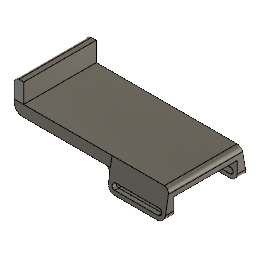
laptop_slider (Autodesk Fusion 360 design; units mm, degrees)
Autodesk Fusion 360 part; units mm, degrees
sketch "Sketch1" plane through (0, 0, 0) normal (0, 0, 1) x (1, 0, 0)
  line L0 (160, 0) -> (160, 10)
  line L1 (160, 10) -> (10, 10)
  line L2 (0, 10) -> (0, 25)
  line L3 (5, 30) -> (10, 30)
  line L4 (10, 30) -> (10, 10)
  arc A0 (5, 30) -> (0, 25) centre (5, 25) ccw
  line L5 (146, 0) -> (146, -12.5)
  line L6 (160, -12.5) -> (160, 0)
  arc A1 (146, -12.5) -> (160, -12.5) centre (153, -12.5) ccw
  line L7 (101, -12.5) -> (101, 0)
  line L8 (115, -12.5) -> (115, 0)
  arc A2 (101, -12.5) -> (115, -12.5) centre (108, -12.5) ccw
  line L9 (10, 0) -> (101, 0)
  line L10 (115, 0) -> (146, 0)
  line L11 (108, -15.5) -> (109.157, -15.2679)
  line L12 (153.0016, -15.5) -> (108, -15.5)
  line L13 (108, -9.5) -> (153, -9.5)
  line L14 (153, -19.5) -> (108, -19.5)
  arc A3 (108, -9.5) -> (109.157, -15.2679) centre (108, -12.5) ccw
  arc A4 (153.0016, -15.5) -> (153, -9.5) centre (153, -12.5) ccw
  arc A5 (0, 10) -> (10, 0) centre (10, 10) ccw
  point P0 (0, 30)
  dimension "d1" = 160
  dimension "d2" = 10
  dimension "d3" = 20
  dimension "d4" = 10
  dimension "d6" = 5
  dimension "d7" = 25
  dimension "d8" = 6
  dimension "d10" = 14
  dimension "d12" = 6
  dimension "d14" = 14
  dimension "d15" = 22.5
  dimension "d16" = 14
  dimension "d31" = 45
  dimension "d45" = 10
  constraint horizontal L9
  constraint vertical L0
  constraint horizontal L1
  constraint perpendicular L1 L2
  constraint perpendicular L2 L3
  constraint perpendicular L1 L4
  constraint coincident origin L9
  constraint coincident P0 L2
  constraint coincident P0 L3
  constraint tangent L2 A0
  constraint tangent L3 A0
  constraint concentric A1 A4
  constraint coincident L5.start L9
  constraint tangent L5 A1
  constraint coincident L0.start L9
  constraint tangent L6 A1
  constraint perpendicular L6 L9
  constraint concentric A2 A3
  constraint perpendicular L7 L9
  constraint coincident L8.end L9
  constraint perpendicular L8 L9
  constraint collinear L9 L10
  constraint coincident L11.start A3
  constraint horizontal L12
  constraint coincident L13.end A4
  constraint tangent L13 A4
  constraint midpoint A1 L14.start
  constraint midpoint A2 L14.end
  constraint coincident L13 A4.end
  constraint tangent L13 A3
  constraint tangent L12 A3
  constraint coincident L0.start L6.end
  constraint tangent L2 A5
  constraint tangent L9 A5
  measures "d1" distance of origin L0.start
  measures "d2" distance of L0.start L0.end
  measures "d3" distance of L2.start P0
  measures "d4" distance of P0 L3.end
  measures "d6" radius of A0
  measures "d7" distance of A0.centre L9
  measures "d8" diameter of A4
  measures "d10" distance of L5 L6
  measures "d12" diameter of A3
  measures "d14" diameter of A2
  measures "d15" distance of L1 A2.centre
  measures "d16" distance of L7 L8
  measures "d31" distance of A1.centre A2.centre
  measures "d45" radius of A5
extrude "Extrude3" add sketch "Sketch1" along normal blind 75 contours L0 L1 L2 L3 L4 A0 L5 L6 A1 L7 L8 A2 L9 L10 L12 L13 A3 A4 A5 | A1 A2 L12 L14 | L5 L8 L10 L13
sketch "Sketch3" plane through (0, -19.5, 0) normal (0, -1, 0) x (1, 0, 0)
  line L0 (108, 0) -> (153, 0)
  line L1 (153, 0) -> (153, 75)
  line L2 (153, 75) -> (108, 75)
  line L3 (108, 75) -> (108, 0)
  line L4 (15, 70) -> (170, 70)
  line L5 (170, 70) -> (170, 5)
  line L6 (170, 5) -> (15, 5)
  line L7 (15, 5) -> (15, 70)
  line L8 (160, 0) -> (160, 75)
  line L9 (5, 0) -> (5, 75)
  dimension "d34" = 5
  dimension "d35" = 5
  dimension "d37" = 10
  dimension "d40" = 10
  constraint horizontal L4
  constraint vertical L5
  constraint horizontal L6
  constraint vertical L7
  measures "d34" distance of L2 L4
  measures "d35" distance of L0 L6
  measures "d37" distance of L7 L9
  measures "d40" distance of L5 L8
extrude "Extrude4" cut sketch "Sketch3" against normal blind 19.5 contours L3 L4 L6 L7 | L1 L3 L4 L6 | L1 L4 L6 L8 | L4 L5 L6 L8
sketch "Sketch4" plane through (10, 0, 0) normal (1, 0, 0) x (0, 1, 0)
  line L0 (10, 0) -> (30, 0)
  line L1 (30, 0) -> (30, 75)
  line L2 (30, 75) -> (10, 75)
  line L3 (10, 75) -> (10, 0)
  line L4 (-19.5, 0) -> (-19.5, -5.0219)
  line L5 (-19.5, -5.0219) -> (10, 0)
  line L6 (-19.5, 0) -> (10, 0)
  line L7 (-19.5, 75) -> (10, 75)
  line L8 (-19.5, 75) -> (-19.5, 80.0219)
  line L9 (-19.5, 80.0219) -> (10, 75)
  dimension "d50" = 9.661
  dimension "d53" = 29.5
  dimension "d55" = 9.661
  dimension "d56" = 29.5
  constraint vertical L4
  constraint coincident L0.start L3.end
  constraint perpendicular L3 L6
  constraint coincident L2.end L3.start
  constraint perpendicular L7 L8
  measures "d50" angle of L5 L6
  measures "d53" distance of L4.start L0.start
  measures "d55" angle of L7 L9
  measures "d56" distance of L7.start L2.end
extrude "Extrude5" add sketch "Sketch4" along normal blind 150 contours L7 L8 L9 | L4 L5 L6
extrude "Extrude6" cut 1 faces at (138.0005, -13.5, 75) along direction (0, 0, 1) blind 50
extrude "Extrude7" cut 1 faces at (138.0005, -13.5, 0) along direction (0, 0, -1) blind 65
extrude "Extrude8" cut 1 faces at (158.6248, -18.1248, 0) along direction (0, 0, -1) blind 11
extrude "Extrude9" cut 1 faces at (158.6248, -18.1248, 75) along direction (0, 0, 1) blind 8
extrude "Extrude10" cut 1 faces at (10, -13, 76.674) along direction (1, 0, 0) blind 90
extrude "Extrude11" cut 1 faces at (10, -13, -1.674) along direction (1, 0, 0) blind 90
extrude "Extrude12" cut 1 faces at (100, -13, -1.674) along direction (1, 0, 0) blind 1
extrude "Extrude13" cut 1 faces at (100, -13, 76.674) along direction (1, 0, 0) blind 1
extrude "Extrude14" cut 1 faces at (102.3752, -18.1248, 0) along direction (0, 0, -1) blind 12
extrude "Extrude15" cut 1 faces at (102.3752, -18.1248, 75) along direction (0, 0, 1) blind 10
sketch "Sketch5" plane through (101, 0, 0) normal (-1, 0, 0) x (0, -1, 0)
  line L0 (12.5, 75) -> (12.5, 78.8302)
  line L1 (12.5, 78.8302) -> (-10, 75)
  line L2 (-10, 75) -> (0, 75)
  line L3 (0, 75) -> (0, 70)
  line L4 (0, 70) -> (12.5, 70)
  line L5 (12.5, 70) -> (12.5, 75)
  line L6 (0, 0) -> (-10, 0)
  line L7 (0, 0) -> (0, -1.7023)
  line L8 (-10, 0) -> (0, -1.7023)
  line L9 (-10, 75) -> (0, 75)
  line L10 (0, 76.7023) -> (0, 75)
  line L11 (0, 76.7023) -> (-10, 75)
  dimension "d79" = 9.661
  dimension "d80" = 10
  dimension "d81" = 9.661
  constraint coincident L6.start L7.start
  constraint horizontal L6
  constraint perpendicular L6 L7
  constraint coincident L1.end L2.start
  constraint coincident L2.end L3.start
  constraint perpendicular L2 L10
  measures "d79" angle of L6 L8
  measures "d80" horizontal distance of L6.end L7.end
  measures "d81" angle of L9 L11
extrude "Extrude16" add sketch "Sketch5" along normal blind 110 contours L1 L2 L9 L10 L11 | L6 L7 L8
extrude "Extrude17" cut 1 faces at (-5.865, 5.7276, 0) along direction (0, 0, -1) blind 10
extrude "Extrude18" cut 1 faces at (-5.865, 5.7276, 75) along direction (0, 0, 1) blind 15
fillet "Fillet4" radius 5 2 edges at (101, 0, 2.5) (101, 0, 72.5)
fillet "Fillet5" radius 5 1 edges at (160, 10, 37.5)
move_body "Move1" bodies 1 to x (1, 0, 0) y (0, 0, 1) z (0, -1, 0) at (0, -21, 21)
equation "d15 = 24 mm - 1.5 mm"
